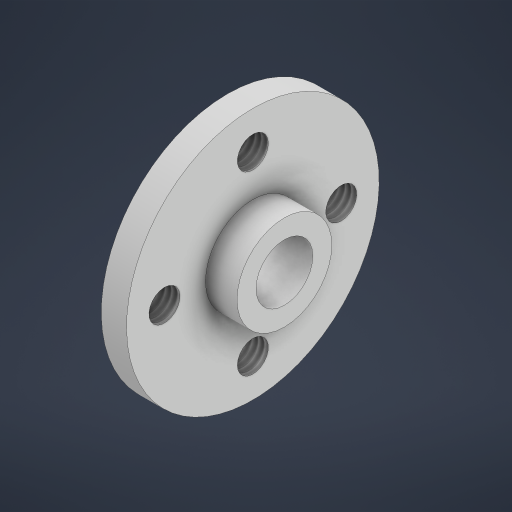
# Autodesk Inventor part: Motor Adapter
Saved by Autodesk Inventor 2024 (Build 280153000, 153)
## iProperties
Created: 2024-02-24
Part Number: Motor Adapter
Material: Generisch
Document SubType Name: Modeling
Designer: jacob
Density: 1 g/cm^3
Appearance: Vorgabe
Author: jacob
Autodesk Inventor part; units mm, degrees
ref_plane "YZ Plane" through (0, 0, 0) normal (1, 0, 0) x (0, 1, 0)
ref_plane "XZ Plane" through (0, 0, 0) normal (0, 1, 0) x (-1, 0, 0)
ref_plane "XY Plane" through (0, 0, 0) normal (0, 0, 1) x (1, 0, 0)
sketch "Skizze1" plane through (0, 0, 0) normal (0, 0, 1) x (1, 0, 0)
  line L0 (0, 0) -> (4.5, 0)
  line L1 (0, 1.5) -> (1, 1.5)
  line L2 (1, 1.5) -> (1, 2.25)
  line L3 (1, 2.25) -> (4.5, 2.25)
  line L4 (4.5, 2.25) -> (4.5, 3.75)
  line L5 (4.5, 3.75) -> (2, 3.75)
  line L6 (2, 3.75) -> (2, 10)
  line L7 (2, 10) -> (0, 10)
  line L8 (0, 10) -> (0, 1.5)
  point P0 (0.5, 1.5)
  dimension "d0" = 4.5
  dimension "d1" = 3
  dimension "d2" = 1
  dimension "d3" = 7.5
  dimension "d4" = 4.5
  dimension "d5" = 2
  dimension "d6" = 20
  constraints: 18 end point, 7 perpendicular, 2 horizontal, 2 vertical alignment, 1 midpoint
  measures "d0" diameter of L3 L0
  measures "d1" diameter of point (0.5, 1.5) L0
  measures "d2" distance of L1.start L1.end
  measures "d3" diameter of L5 L0
  measures "d4" distance between parallel lines of L8 L4
  measures "d5" distance of L6.end L7.end
  measures "d6" diameter of L7 L0
revolve "Umdrehung1" add sketch "Skizze1" angle 360 about axis through (0, 0, 0) along (1, 0, 0)
sketch "Skizze2" plane through (2, 0, 0) normal (1, 0, 0) x (0, 0, -1)
  point P0 (0, 0)
  point P1 (0, 7)
  dimension "d8" = 7
  constraints: 1 vertical alignment
  measures "d8" distance of point (0, 7) point (0, 0)
hole "Bohrung1" at (2, 7, 0) direction (-1, 0, 0) diameter 2.459 end through all thread size "M3x0.5" class "6H" standard "ISO Metric profile"
pattern_circular "Runde Anordnung1" count 4 over 360 about axis through (2.75, 0, 0) along (1, 0, 0) of "Bohrung1"
